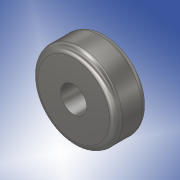
# Autodesk Inventor part: 14x4x4mm Bearing
Saved by Autodesk Inventor 2017 (Build 210142000, 142)
## iProperties
Created: 2017-07-05
Part Number: 14x4x4mm Bearing
Material: Steel, Carbon
Document SubType Name: Modeling
Designer: zallen
Density: 7.85 g/cm^3
Appearance: Semi-Polished
Author: zallen
Autodesk Inventor part; units mm, degrees
ref_plane "YZ Plane" through (0, 0, 0) normal (1, 0, 0) x (0, 1, 0)
ref_plane "XZ Plane" through (0, 0, 0) normal (0, 1, 0) x (-1, 0, 0)
ref_plane "XY Plane" through (0, 0, 0) normal (0, 0, 1) x (1, 0, 0)
sketch "Sketch1" plane through (0, 0, 0) normal (0, 0, 1) x (1, 0, 0)
  circle A0 centre (0, 0) radius 6.5
  circle A1 centre (0, 0) radius 2
  dimension "d0" = 13
  dimension "d1" = 4
  constraints: 2 centre point, 2 coincident
  measures "d0" diameter of A0
  measures "d1" diameter of A1
extrude "Extrusion1" add sketch "Sketch1" along normal blind 5
fillet "Fillet1" radius 1 2 edges at (-6.5, 0, 5) (-6.5, 0, 0)
body "Solid1"
